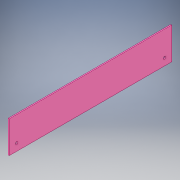
# Autodesk Inventor part: inner_wall
Saved by Autodesk Inventor 2017 (Build 210142000, 142)
## iProperties
Created: 2017-11-22
Part Number: inner_wall
Material: Generic
Document SubType Name: Modeling
Designer: guirguk
Density: 1 g/cm^3
Appearance: Pink
Author: guirguk
Autodesk Inventor part; units mm, degrees
ref_plane "YZ Plane" through (0, 0, 0) normal (1, 0, 0) x (0, 1, 0)
ref_plane "XZ Plane" through (0, 0, 0) normal (0, 1, 0) x (-1, 0, 0)
ref_plane "XY Plane" through (0, 0, 0) normal (0, 0, 1) x (1, 0, 0)
sketch "Sketch1" plane through (0, 0, 0) normal (1, 0, 0) x (0, 1, 0)
  line L0 (0, 0) -> (0, -501.65)
  line L1 (0, -501.65) -> (98.425, -501.65)
  line L2 (98.425, -501.65) -> (98.425, 0)
  line L3 (98.425, 0) -> (0, 0)
  dimension "d0" = 501.65
  dimension "d1" = 98.425
  constraints: 8 end point, 3 perpendicular, 1 vertical
  measures "d0" distance of L0.start L0.end
  measures "d1" distance of L0.end L1.end
extrude "Extrusion1" add sketch "Sketch1" along normal blind 3.175
sketch "Sketch2" plane through (3.175, 0, 0) normal (1, 0, 0) x (0, 0, -1)
  line L0 (0, 0) -> (501.65, 0) projected
  line L1 (0, 0) -> (0, 22.225)
  line L2 (0, 98.425) -> (0, 0) projected
  line L3 (0, 22.225) -> (22.225, 22.225)
  circle A0 centre (22.225, 22.225) radius 3.9687
  dimension "d4" = 22.225
  dimension "d5" = 22.225
  dimension "d6" = 7.9375
  constraints: 4 end point, 1 centre point, 1 coincident, 1 perpendicular, 1 point on line
  measures "d4" distance of L0.start L1.end
  measures "d5" distance of L1.end L3.end
  measures "d6" diameter of A0
extrude "Extrusion2" cut sketch "Sketch2" against normal blind 3.175
sketch "Sketch3" plane through (3.175, 0, 0) normal (1, 0, 0) x (0, 0, -1)
  line L0 (501.65, 0) -> (501.65, 98.425) projected
  line L1 (501.65, 0) -> (501.65, 22.225)
  line L2 (501.65, 22.225) -> (479.425, 22.225)
  circle A0 centre (479.425, 22.225) radius 3.9688
  point P0 (0, 0)
  dimension "d11" = 22.225
  dimension "d12" = 22.225
  dimension "d13" = 7.9375
  constraints: 4 end point, 1 centre point, 1 coincident, 1 perpendicular, 1 point on line
  measures "d11" distance of L0.start L1.end
  measures "d12" distance of L1.end L2.end
  measures "d13" diameter of A0
extrude "Extrusion3" cut sketch "Sketch3" against normal blind 3.175
body "Solid1"
